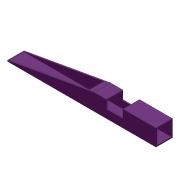
# Autodesk Inventor part: Shovel_BottomFrame
Saved by Autodesk Inventor 2012 (Build 160160000, 160)
## iProperties
Created: 2013-01-29
Part Number: Shovel_BottomFrame
Material: Aluminum-6061
Document SubType Name: Modeling
Designer: JesseK
Density: 2.71 g/cm^3
Mass: 62.4983 g
Surface Area: 300.948 cm^2
Volume: 23.0621 cm^3
Author: JesseK
Autodesk Inventor part; units mm, degrees
ref_plane "YZ Plane" through (0, 0, 0) normal (1, 0, 0) x (0, 1, 0)
ref_plane "XZ Plane" through (0, 0, 0) normal (0, 1, 0) x (-1, 0, 0)
ref_plane "XY Plane" through (0, 0, 0) normal (0, 0, 1) x (1, 0, 0)
sketch "Sketch1" plane through (0, 0, 0) normal (0, 0, 1) x (1, 0, 0)
  line L0 (0, 0) -> (-228.6, 0)
  line L1 (-228.6, 0) -> (-228.6, 1.5875)
  line L2 (-228.6, 1.5875) -> (-95.25, 25.4)
  line L3 (-95.25, 25.4) -> (0, 25.4)
  line L4 (0, 25.4) -> (0, 0)
  dimension "d0" = 25.4
  dimension "d1" = 228.6
  dimension "d2" = 1.5875
  dimension "d3" = 95.25
  constraints: 10 end point, 2 horizontal, 2 vertical
  measures "d0" distance of L3.end L0.start
  measures "d1" distance of L0.start L0.end
  measures "d2" distance of L0.end L1.end
  measures "d3" distance of L2.end L3.end
extrude "Extrusion1" add sketch "Sketch1" along normal blind 25.4
shell "Shell1" thickness 1.5875 removed faces 2 at (-184.15, 9.525, 8.4667) at (0, 16.9333, 8.4667)
sketch "Sketch2" plane through (0, 0, 0) normal (0, 0, -1) x (-1, 0, 0)
  line L0 (95.25, 25.4) -> (0, 25.4) projected
  line L1 (0, 25.4) -> (0, 0) projected
  line L2 (50.8, 25.4) -> (76.2, 25.4)
  line L3 (76.2, 25.4) -> (76.2, 12.7)
  line L4 (76.2, 12.7) -> (50.8, 12.7)
  line L5 (50.8, 12.7) -> (50.8, 25.4)
  dimension "d7" = 25.4
  dimension "d8" = 12.7
  dimension "d9" = 50.8
  constraints: 8 end point, 2 parallel, 1 horizontal, 1 perpendicular, 1 point on line
  measures "d7" distance of L3.end L4.end
  measures "d8" distance of L4.end L2.start
  measures "d9" distance between parallel lines of L5 L1
extrude "Extrusion2" cut sketch "Sketch2" against normal through all
body "Solid1"
